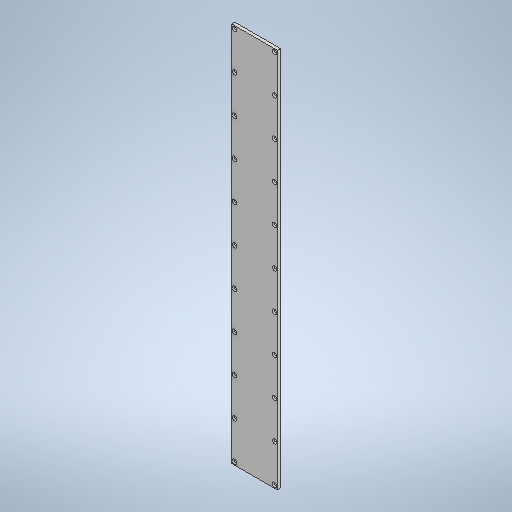
# Autodesk Inventor part: Unterer_Deckel
Saved by Autodesk Inventor 2025.2 (Build 292293000, 293)
## iProperties
Created: 2025-01-07
Part Number: Unterer_Deckel
Material: Generisch
Document SubType Name: Modeling
Designer: gorenfl4
Density: 1 g/cm^3
Appearance: Vorgabe
Author: gorenfl4
Autodesk Inventor part; units mm, degrees
ref_plane "YZ Plane" through (0, 0, 0) normal (1, 0, 0) x (0, 1, 0)
ref_plane "XZ Plane" through (0, 0, 0) normal (0, 1, 0) x (-1, 0, 0)
ref_plane "XY Plane" through (0, 0, 0) normal (0, 0, 1) x (1, 0, 0)
sketch "Skizze1" plane through (0, 0, 0) normal (0, 1, 0) x (-1, 0, 0)
  line L0 (22.9029, 192.7834) -> (-37.0971, 192.7834)
  line L1 (-37.0971, 192.7834) -> (-37.0971, -307.2166)
  line L2 (-37.0971, -307.2166) -> (22.9029, -307.2166)
  line L3 (22.9029, -307.2166) -> (22.9029, 192.7834)
  dimension "d15" = 500
  dimension "d16" = 60
  constraints: 8 end point, 2 parallel, 1 horizontal, 1 perpendicular
  measures "d15" distance between parallel lines of L2 L0
  measures "d16" distance between parallel lines of L1 L3
extrude "Extrusion1" add sketch "Skizze1" along normal blind 4
sketch "Skizze3" plane through (0, 0, 0) normal (0, -1, 0) x (1, 0, 0)
  line L0 (-22.9029, 192.7834) -> (37.0971, 192.7834) projected
  line L1 (-22.9029, -307.2166) -> (-22.9029, 192.7834) projected
  point P0 (0, 0)
  point P1 (-19.1529, 188.7834)
  dimension "d74" = 4
  dimension "d75" = 3.75
  measures "d74" distance from line of L0 point (-19.153, 188.783)
  measures "d75" distance from line of L1 point (-19.153, 188.783)
hole "Bohrung1" at (-19.1529, 0, 188.7834) direction (0, 1, 0) diameter 3 end through all countersink diameter 6 countersink angle 90
pattern_linear "Rechteckige Anordnung1" count 11 spacing 49.2 along (0, 0, -1) count 2 spacing 52.5 along (1, 0, 0) of "Bohrung1"
